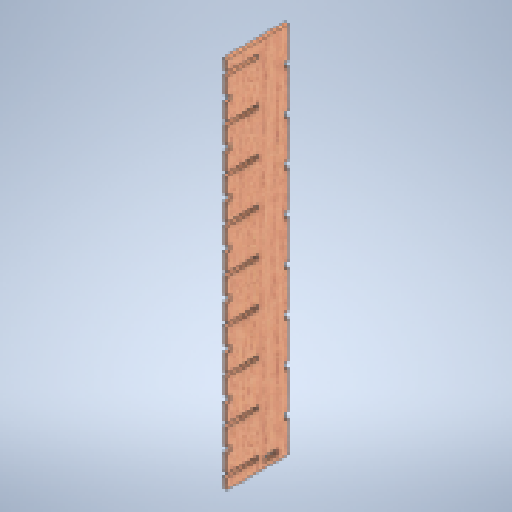
# Autodesk Inventor part: Separators
Saved by Autodesk Inventor 2024 (Build 280153000, 153)
## iProperties
Created: 2023-07-19
Part Number: Separators
Material: Generic
Document SubType Name: Modeling
Designer: Bruno
Density: 1 g/cm^3
Appearance: Default
Author: Bruno
Autodesk Inventor part; units mm, degrees
ref_plane "YZ Plane" through (0, 0, 0) normal (1, 0, 0) x (0, 1, 0)
ref_plane "XZ Plane" through (0, 0, 0) normal (0, 1, 0) x (-1, 0, 0)
ref_plane "XY Plane" through (0, 0, 0) normal (0, 0, 1) x (1, 0, 0)
sketch "Sketch1" plane through (0, 0, 0) normal (1, 0, 0) x (0, 1, 0)
  line L0 (8.45, 60) -> (8.45, 30)
  line L1 (8.45, 30) -> (10, 30)
  line L2 (10, 30) -> (11.55, 30)
  line L3 (11.55, 30) -> (11.55, 60)
  line L4 (11.55, 60) -> (25, 60)
  line L5 (25, 60) -> (25, 57)
  line L6 (25, 57) -> (30, 57)
  line L7 (30, 57) -> (30, 60)
  line L8 (30, 60) -> (43.45, 60)
  line L9 (43.45, 60) -> (43.45, 30)
  line L10 (43.45, 30) -> (45, 30)
  line L11 (10, 0) -> (25, 0)
  line L12 (25, 0) -> (25, 3)
  line L13 (25, 3) -> (30, 3)
  line L14 (30, 3) -> (30, 0)
  line L15 (30, 0) -> (45, 0)
  line L16 (45, 30) -> (46.55, 30)
  line L17 (46.55, 30) -> (46.55, 60)
  line L18 (46.55, 60) -> (60, 60)
  line L19 (60, 57) -> (65, 57)
  line L20 (60, 60) -> (60, 57)
  line L21 (65, 57) -> (65, 60)
  line L22 (65, 60) -> (78.45, 60)
  line L23 (78.45, 60) -> (78.45, 30)
  line L24 (78.45, 30) -> (80, 30)
  line L25 (65, 0) -> (80, 0)
  line L26 (60, 3) -> (65, 3)
  line L27 (65, 3) -> (65, 0)
  line L28 (60, 0) -> (60, 3)
  line L29 (45, 0) -> (60, 0)
  line L30 (80, 30) -> (81.55, 30)
  line L31 (81.55, 30) -> (81.55, 60)
  line L32 (81.55, 60) -> (95, 60)
  line L33 (95, 57) -> (100, 57)
  line L34 (95, 60) -> (95, 57)
  line L35 (100, 57) -> (100, 60)
  line L36 (100, 60) -> (113.45, 60)
  line L37 (113.45, 60) -> (113.45, 30)
  line L38 (113.45, 30) -> (115, 30)
  line L39 (100, 0) -> (115, 0)
  line L40 (95, 3) -> (100, 3)
  line L41 (100, 3) -> (100, 0)
  line L42 (95, 0) -> (95, 3)
  line L43 (80, 0) -> (95, 0)
  line L44 (115, 30) -> (116.55, 30)
  line L45 (116.55, 30) -> (116.55, 60)
  line L46 (116.55, 60) -> (130, 60)
  line L47 (130, 57) -> (135, 57)
  line L48 (130, 60) -> (130, 57)
  line L49 (135, 57) -> (135, 60)
  line L50 (135, 60) -> (148.45, 60)
  line L51 (148.45, 60) -> (148.45, 30)
  line L52 (148.45, 30) -> (150, 30)
  line L53 (135, 0) -> (150, 0)
  line L54 (130, 3) -> (135, 3)
  line L55 (135, 3) -> (135, 0)
  line L56 (130, 0) -> (130, 3)
  line L57 (115, 0) -> (130, 0)
  line L58 (150, 30) -> (151.55, 30)
  line L59 (151.55, 30) -> (151.55, 60)
  line L60 (151.55, 60) -> (165, 60)
  line L61 (165, 57) -> (170, 57)
  line L62 (165, 60) -> (165, 57)
  line L63 (170, 57) -> (170, 60)
  line L64 (170, 60) -> (183.45, 60)
  line L65 (183.45, 60) -> (183.45, 30)
  line L66 (183.45, 30) -> (185, 30)
  line L67 (170, 0) -> (185, 0)
  line L68 (165, 3) -> (170, 3)
  line L69 (170, 3) -> (170, 0)
  line L70 (165, 0) -> (165, 3)
  line L71 (150, 0) -> (165, 0)
  line L72 (185, 30) -> (186.55, 30)
  line L73 (186.55, 30) -> (186.55, 60)
  line L74 (186.55, 60) -> (200, 60)
  line L75 (200, 57) -> (205, 57)
  line L76 (200, 60) -> (200, 57)
  line L77 (205, 57) -> (205, 60)
  line L78 (205, 60) -> (218.45, 60)
  line L79 (218.45, 60) -> (218.45, 30)
  line L80 (218.45, 30) -> (220, 30)
  line L81 (205, 0) -> (220, 0)
  line L82 (200, 3) -> (205, 3)
  line L83 (205, 3) -> (205, 0)
  line L84 (200, 0) -> (200, 3)
  line L85 (185, 0) -> (200, 0)
  line L86 (220, 30) -> (221.55, 30)
  line L87 (221.55, 30) -> (221.55, 60)
  line L88 (221.55, 60) -> (235, 60)
  line L89 (235, 57) -> (240, 57)
  line L90 (235, 60) -> (235, 57)
  line L91 (240, 57) -> (240, 60)
  line L92 (240, 60) -> (253.45, 60)
  line L93 (253.45, 60) -> (253.45, 30)
  line L94 (253.45, 30) -> (255, 30)
  line L95 (240, 0) -> (255, 0)
  line L96 (235, 3) -> (240, 3)
  line L97 (240, 3) -> (240, 0)
  line L98 (235, 0) -> (235, 3)
  line L99 (220, 0) -> (235, 0)
  line L100 (255, 30) -> (256.55, 30)
  line L101 (256.55, 30) -> (256.55, 60)
  line L102 (256.55, 60) -> (270, 60)
  line L103 (270, 57) -> (275, 57)
  line L104 (270, 60) -> (270, 57)
  line L105 (275, 57) -> (275, 60)
  line L106 (275, 60) -> (288.45, 60)
  line L107 (288.45, 60) -> (288.45, 30)
  line L108 (288.45, 30) -> (290, 30)
  line L109 (275, 0) -> (290, 0)
  line L110 (270, 3) -> (275, 3)
  line L111 (275, 3) -> (275, 0)
  line L112 (270, 0) -> (270, 3)
  line L113 (255, 0) -> (270, 0)
  line L114 (150, 0) -> (150, 30) construction
  line L115 (8.45, 0) -> (10, 0)
  line L116 (0, 60) -> (8.45, 60)
  line L117 (0, 0) -> (10, 0)
  line L118 (300, 60) -> (300, 0)
  line L119 (291.55, 60) -> (291.55, 30)
  line L120 (291.55, 30) -> (290, 30)
  line L121 (291.55, 0) -> (290, 0)
  line L122 (300, 60) -> (291.55, 60)
  line L123 (300, 0) -> (290, 0)
  line L124 (0, 0) -> (0, 60)
  line L125 (4.45, 10) -> (8.45, 10)
  line L126 (8.45, 10) -> (8.45, 20)
  line L127 (8.45, 20) -> (4.45, 20)
  line L128 (4.45, 20) -> (4.45, 10)
  point P0 (9.225, 30)
  point P1 (290.775, 30)
  point P2 (300, 0)
  dimension "d36" = 1.55
  dimension "d37" = 1.55
  dimension "d39" = 5
  dimension "d41" = 1.55
  dimension "d42" = 35
  dimension "d43" = 5
  dimension "d45" = 3
  dimension "d46" = 35
  dimension "d51" = 35
  dimension "d61" = 30
  dimension "d62" = 60
  dimension "d63" = 3
  dimension "d69" = 8.45
  dimension "d74" = 10
  dimension "d75" = 4
  dimension "d76" = 10
  constraints: 258 end point, 48 point on line, 12 perpendicular, 8 symmetric about line, 5 horizontal, 4 collinear, 4 vertical alignment, 3 parallel, 2 vertical, 1 coincident, 1 horizontal alignment, 1 midpoint, 209 other
  measures "d36" distance of L0.end L1.end
  measures "d37" distance of L1.end L2.end
  measures "d39" distance of L5.end L6.end
  measures "d41" distance of L9.end L10.end
  measures "d42" distance of L10.end L1.end
  measures "d43" distance of L12.end L13.end
  measures "d45" distance of L11.end L12.end
  measures "d46" distance of L11.start L15.end
  measures "d51" distance of L2.end L16.end
  measures "d61" distance from line of L4 point (9.225, 30)
  measures "d62" distance between parallel lines of L11 L4
  measures "d63" distance of L6.end L7.end
  measures "d69" distance of L116.start L0.start
  measures "d74" distance of L125.end L126.end
  measures "d75" distance of L125.start L125.end
  measures "d76" distance from line of L117 L125.start
extrude "Extrusion1" add sketch "Sketch1" along normal blind 3
body "Solid1"
